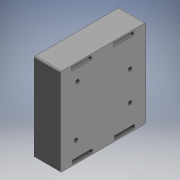
# Autodesk Inventor part: frame_top
Saved by Autodesk Inventor 2016 (Build 200138000, 138)
## iProperties
Created: 2017-09-13
Part Number: frame_top
Material: Generic
Document SubType Name: Modeling
Designer: Student
Density: 1 g/cm^3
Appearance: Default
Author: Student
Autodesk Inventor part; units mm, degrees
ref_plane "YZ Plane" through (0, 0, 0) normal (1, 0, 0) x (0, 1, 0)
ref_plane "XZ Plane" through (0, 0, 0) normal (0, 1, 0) x (-1, 0, 0)
ref_plane "XY Plane" through (0, 0, 0) normal (0, 0, 1) x (1, 0, 0)
sketch "Sketch1" plane through (0, 0, 0) normal (1, 0, 0) x (0, 1, 0)
  line L0 (46.6598, -89.1794) -> (0, -89.1794)
  line L1 (46.6598, -89.1794) -> (37.8968, -89.1794)
  line L2 (30.0736, -89.1794) -> (24.6634, -89.1794)
  line L3 (64.4398, -89.1794) -> (46.6598, -89.1794)
  line L4 (0, -89.1794) -> (-12.7, -89.1794)
  line L5 (-17.78, -6.35) -> (64.4398, -6.35)
  circle A0 centre (5.9286, -73.66) radius 1.651
  circle A1 centre (34.3662, -73.66) radius 1.651
  circle A2 centre (0.8486, -21.336) radius 1.651
  circle A3 centre (49.3626, -22.86) radius 1.651
  line L6 (-12.7, -89.1794) -> (-17.78, -89.1794)
  line L7 (-19.05, -87.9094) -> (-19.05, -7.62)
  line L8 (65.7098, -87.9094) -> (65.7098, -7.62)
  line L9 (61.1505, -76.9747) -> (61.1505, -57.8485)
  line L10 (61.1505, -57.8485) -> (64.1985, -57.8485)
  line L11 (64.1985, -57.8485) -> (64.1985, -76.9747)
  line L12 (64.1985, -76.9747) -> (61.1505, -76.9747)
  line L13 (61.1505, -36.1823) -> (61.1505, -17.0561)
  line L14 (61.1505, -17.0561) -> (64.1985, -17.0561)
  line L15 (64.1985, -17.0561) -> (64.1985, -36.1823)
  line L16 (64.1985, -36.1823) -> (61.1505, -36.1823)
  line L17 (-17.2028, -77.8891) -> (-17.2028, -58.7629)
  line L18 (-17.2028, -58.7629) -> (-14.1548, -58.7629)
  line L19 (-14.1548, -58.7629) -> (-14.1548, -77.8891)
  line L20 (-14.1548, -77.8891) -> (-17.2028, -77.8891)
  line L21 (-17.2593, -37.0967) -> (-17.2593, -17.9705)
  line L22 (-17.2593, -17.9705) -> (-14.2113, -17.9705)
  line L23 (-14.2113, -17.9705) -> (-14.2113, -37.0967)
  line L24 (-14.2113, -37.0967) -> (-17.2593, -37.0967)
  arc A4 (65.7098, -7.62) -> (64.4398, -6.35) centre (64.4398, -7.62) ccw
  arc A5 (-17.78, -6.35) -> (-19.05, -7.62) centre (-17.78, -7.62) ccw
  arc A6 (-19.05, -87.9094) -> (-17.78, -89.1794) centre (-17.78, -87.9094) ccw
  arc A7 (64.4398, -89.1794) -> (65.7098, -87.9094) centre (64.4398, -87.9094) ccw
  point P0 (65.7098, -89.1794)
  point P1 (24.6634, -89.1794)
  point P2 (-19.05, -89.1794)
  point P3 (-19.05, -6.35)
  dimension "d50" = 5.08
  dimension "d53" = 25.4
  dimension "d87" = 82.8294
  dimension "d90" = 3.302
  dimension "d98" = 3.302
  dimension "d102" = 6.35
  dimension "d104" = 19.1262
  dimension "d108" = 19.1262
  dimension "d109" = 3.048
  dimension "d110" = 19.1262
  dimension "d114" = 19.1262
  dimension "d115" = 3.048
  dimension "d126" = 21.6662
  dimension "d127" = 3.048
  dimension "d128" = 3.048
  dimension "d129" = 21.6662
  dimension "d130" = 1.27
  constraints: 50 end point, 8 centre point, 8 parallel, 8 point on circle, 8 point on line, 8 tangent, 5 perpendicular, 4 vertical, 3 equal radius, 3 horizontal
  measures "d87" distance between parallel lines of L3 L5
  measures "d90" diameter of A1
  measures "d98" diameter of A3
  measures "d102" distance of point (-19.05, -89.179) L4.end
  measures "d104" distance of L9.start L9.end
  measures "d108" distance of L13.start L14.start
  measures "d109" distance of L14.start L14.end
  measures "d110" distance of L20.end L17.end
  measures "d114" distance of L24.end L21.end
  measures "d115" distance of L21.end L23.start
  measures "d126" distance between parallel lines of L10 L16
  measures "d127" distance of L11.end L9.start
  measures "d128" distance of L20.start L20.end
  measures "d129" distance between parallel lines of L18 L24
  measures "d130" radius of A4
extrude "Extrusion5" add sketch "Sketch1" along normal blind 25.4
body "Solid5"
